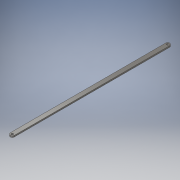
# Autodesk Inventor part: steeringlinkage
Saved by Autodesk Inventor 2018 (Build 220112000, 112)
## iProperties
Created: 2018-08-06
Part Number: steeringlinkage
Material: Steel, Mild
Document SubType Name: Modeling
Designer: Cole Tucker
Density: 7.85 g/cm^3
Appearance: Semi-Polished
Mass: 368.899 g
Surface Area: 203.999 cm^2
Volume: 46.9936 cm^3
Author: Cole Tucker
Autodesk Inventor part; units mm, degrees
ref_plane "YZ Plane" through (0, 0, 0) normal (1, 0, 0) x (0, 1, 0)
ref_plane "XZ Plane" through (0, 0, 0) normal (0, 1, 0) x (-1, 0, 0)
ref_plane "XY Plane" through (0, 0, 0) normal (0, 0, 1) x (1, 0, 0)
sketch "Sketch1" plane through (0, 0, 0) normal (0, 1, 0) x (-1, 0, 0)
  arc A0 (9.525, 0) -> (0, -9.525) centre (0, 0) ccw
  line L0 (0, 0) -> (0, -696.722) construction
  arc A1 (0, -687.197) -> (9.525, -696.722) centre (0, -696.722) ccw
  line L1 (9.525, -696.722) -> (9.525, 0)
  line L2 (-9.525, 0) -> (-9.525, -696.722)
  circle A2 centre (0, -696.722) radius 4.7625
  circle A3 centre (0, 0) radius 4.7625
  dimension "d0" = 19.05
  dimension "d2" = 19.05
  dimension "d3" = 9.525
  dimension "d4" = 9.525
  dimension "d10" = 696.722
  constraints: 6 end point, 6 point on circle, 4 centre point, 4 coincident, 2 point on line, 2 vertical, 1 tangent
  measures "d0" diameter of A0
  measures "d2" diameter of A1
  measures "d3" diameter of A2
  measures "d4" diameter of A3
  measures "d10" distance of L0.start L0.end
extrude "Extrusion2" add sketch "Sketch1" along normal blind 6.35
body "Solid2"
